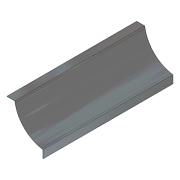
# Autodesk Inventor part: Panel_FrontVerticalConveyorShroud_Lower
Saved by Autodesk Inventor 2012 (Build 160160000, 160)
## iProperties
Created: 2012-01-21
Part Number: Panel_FrontVerticalConveyorShroud_Lower
Material: Polycarbonate, Smoke
Document SubType Name: Modeling
Designer: JesseK
Mass: 141.761 g
Surface Area: 1509.22 cm^2
Volume: 118.134 cm^3
Density: 1.2 g/cm^3
Author: JesseK
Autodesk Inventor part; units mm, degrees
ref_plane "YZ Plane" through (0, 0, 0) normal (1, 0, 0) x (0, 1, 0)
ref_plane "XZ Plane" through (0, 0, 0) normal (0, 1, 0) x (-1, 0, 0)
ref_plane "XY Plane" through (0, 0, 0) normal (0, 0, 1) x (1, 0, 0)
sketch "Sketch1" plane through (0, 0, 0) normal (0, 0, 1) x (1, 0, 0)
  arc A0 (-99.9121, -18.4428) -> (-18.4428, -99.9121) centre (0, 0) ccw
  arc A1 (-102.1936, -14.2875) -> (-14.2875, -102.1936) centre (0, 0) ccw
  line L0 (-99.9121, -18.4428) -> (-100.9721, -12.7)
  line L1 (-100.9721, -12.7) -> (-126.3721, -12.7)
  line L2 (-126.3721, -12.7) -> (-126.3721, -14.2875)
  line L3 (-126.3721, -14.2875) -> (-102.1936, -14.2875)
  line L4 (-18.4428, -99.9121) -> (-12.7, -100.9721)
  line L5 (-12.7, -100.9721) -> (-12.7, -126.3721)
  line L6 (-12.7, -126.3721) -> (-14.2875, -126.3721)
  line L7 (-14.2875, -126.3721) -> (-14.2875, -102.1936)
  line L8 (-132.6152, 0) -> (-97.9265, 0) construction
  line L9 (-97.9265, 0) -> (-97.9265, -12.7) construction
  line L10 (-97.9265, -12.7) -> (-132.6152, -12.7) construction
  line L11 (-132.6152, -12.7) -> (-132.6152, 0) construction
  line L12 (0, -100.3613) -> (-12.7, -100.3613) construction
  line L13 (-12.7, -100.3613) -> (-12.7, -135.05) construction
  line L14 (-12.7, -135.05) -> (0, -135.05) construction
  line L15 (0, -135.05) -> (0, -100.3613) construction
  line L16 (0, -100.3613) -> (0, 0) construction
  line L17 (0, 0) -> (-97.9265, 0) construction
  point P0 (-48.9633, 0)
  dimension "d0" = 1.5875
  dimension "d1" = 1.5875
  dimension "d2" = 101.6
  dimension "d3" = 25.4
  dimension "d6" = 12.7
  constraints: 36 end point, 7 perpendicular, 5 parallel, 4 horizontal, 4 point on circle, 2 centre point, 2 coincident, 2 collinear, 2 tangent, 2 vertical, 1 midpoint
  measures "d0" radial gap between concentric circles of A1 A0
  measures "d1" distance between parallel lines of L5 L7
  measures "d2" radius of A0
  measures "d3" distance of L0.end L1.end
  measures "d6" distance of L8.end L9.end
extrude "Extrusion1" add sketch "Sketch1" along normal blind 406.4
body "Solid1"
